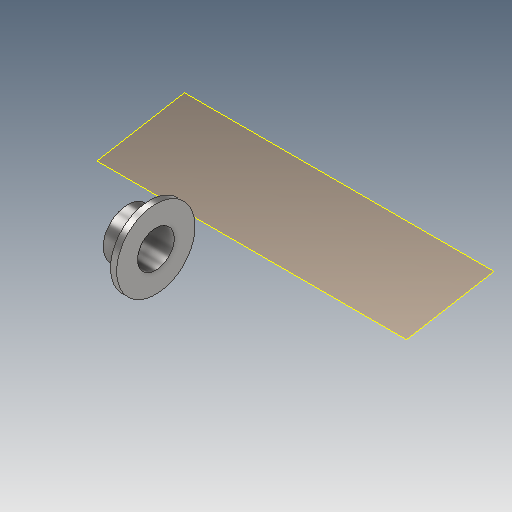
# Autodesk Inventor part: 中间轴套筒
Saved by Autodesk Inventor 2025 (Build 290162000, 162)
## iProperties
Created: 2025-03-20
Part Number: 中间轴套筒
Material: 钢，软
Document SubType Name: Modeling
Designer: liukan
Density: 7.85 g/cm^3
Appearance: 半抛光
Author: liukan
Autodesk Inventor part; units mm, degrees
ref_plane "YZ Plane" through (0, 0, 0) normal (1, 0, 0) x (0, 1, 0)
ref_plane "XZ Plane" through (0, 0, 0) normal (0, 1, 0) x (-1, 0, 0)
ref_plane "XY Plane" through (0, 0, 0) normal (0, 0, 1) x (1, 0, 0)
ref_plane "工作平面1" through (135.5371, 153.7824, 23.3647) normal (0, 0.9849, 0.1733) x (-1, 0, 0)
sketch "草图1" plane through (135.5371, 153.7824, 23.3647) normal (0, 0.9849, 0.1733) x (-1, 0, 0)
  line L0 (-46.1712, 85.482) -> (-46.1712, 53.282) projected
  line L1 (-46.1712, 47.032) -> (-46.1712, 91.732) projected
  line L2 (-72.1712, 92.382) -> (-72.1712, 46.382) projected
  line L3 (-72.1712, 54.382) -> (-72.1712, 84.382) projected
  line L4 (-72.1712, 84.382) -> (-46.1712, 84.382)
  line L5 (-46.1712, 84.382) -> (-46.1712, 89.382)
  line L6 (-46.1712, 89.382) -> (-69.1712, 89.382)
  line L7 (-69.1712, 89.382) -> (-69.1712, 84.382)
  line L8 (-46.1712, 69.382) -> (-72.1712, 69.382)
  line L9 (-69.1712, 43.382) -> (-69.1712, 95.382) projected
  line L10 (-69.1712, 89.382) -> (-64.1712, 89.382)
  line L11 (-64.1712, 89.382) -> (-64.1712, 101.382)
  line L12 (-64.1712, 101.382) -> (-69.1712, 101.382)
  line L13 (-69.1712, 101.382) -> (-69.1712, 89.382)
  point P0 (135.5371, 3.6411)
  point P1 (-71.1712, 89.382)
  point P2 (-69.1712, 69.382)
  dimension "d0" = 20
  dimension "d2" = 5
  dimension "d3" = 12
  constraints: 18 end point, 4 parallel, 4 point on line, 2 horizontal, 2 midpoint, 2 perpendicular
  measures "d0" distance between parallel lines of L8 L6
  measures "d2" distance of L12.end L11.end
  measures "d3" distance of L11.end L10.end
revolve "旋转1" add sketch "草图1" angle 360 about axis through (181.7084, 141.7577, 91.6967) along (1, 0, 0) contours L0 L4 L7 L6 L1 | L6 L9 L13 L12 L11
